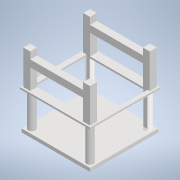
# Autodesk Inventor part: tABLE
Saved by Autodesk Inventor 2021 (Build 250183000, 183)
## iProperties
Created: 2021-06-23
Part Number: tABLE
Material: Brick, Common, Brown
Document SubType Name: Modeling
Designer: user
Density: 1.95 g/cm^3
Appearance: Default
Author: user
Autodesk Inventor part; units mm, degrees
ref_plane "YZ Plane" through (0, 0, 0) normal (1, 0, 0) x (0, 1, 0)
ref_plane "XZ Plane" through (0, 0, 0) normal (0, 1, 0) x (-1, 0, 0)
ref_plane "XY Plane" through (0, 0, 0) normal (0, 0, 1) x (1, 0, 0)
sketch "Sketch6" plane through (0, 0, 0) normal (0, 1, 0) x (-1, 0, 0)
  line L0 (-10, -10) -> (10, -10)
  line L1 (10, -10) -> (10, 10)
  line L2 (10, 10) -> (-10, 10)
  line L3 (-10, 10) -> (-10, -10)
  line L4 (-10, -10) -> (10, 10) construction
  line L5 (10, -10) -> (-10, 10) construction
  point P0 (0, 0)
  dimension "d28" = 20
  dimension "d29" = 20
  constraints: 12 end point, 2 midpoint, 2 parallel, 1 horizontal, 1 perpendicular
  measures "d28" distance of L2.end L1.end
  measures "d29" distance of L1.end L0.end
extrude "Extrusion6" add sketch "Sketch6" along normal blind 1
sketch "Sketch7" plane through (0, 1, 0) normal (0, 1, 0) x (1, 0, 0)
  circle A0 centre (-8.5, -8.5) radius 1
  line L0 (-10, 10) -> (-10, -10) projected
  line L1 (-10, -10) -> (10, -10) projected
  point P0 (0, 0)
  dimension "d32" = 2
  dimension "d33" = 0.5
  dimension "d34" = 0.5
  constraints: 1 centre point
  measures "d32" diameter of A0
  measures "d33" distance edge to line of A0 L0
  measures "d34" distance edge to line of A0 L1
extrude "Extrusion7" add sketch "Sketch7" along normal blind 10
sketch "Sketch8" plane through (0, 1, 0) normal (0, 1, 0) x (1, 0, 0)
  circle A0 centre (-8.5, 8.5) radius 1
  line L0 (-10, 10) -> (-10, -10) projected
  line L1 (10, 10) -> (-10, 10) projected
  point P0 (0, 0)
  dimension "d37" = 2
  dimension "d38" = 0.5
  dimension "d39" = 0.5
  constraints: 1 centre point
  measures "d37" diameter of A0
  measures "d38" distance edge to line of A0 L0
  measures "d39" distance edge to line of A0 L1
extrude "Extrusion8" add sketch "Sketch8" along normal blind 10
sketch "Sketch9" plane through (0, 1, 0) normal (0, 1, 0) x (1, 0, 0)
  circle A0 centre (8.5, -8.5) radius 1
  line L0 (10, -10) -> (10, 10) projected
  line L1 (-10, -10) -> (10, -10) projected
  point P0 (0, 0)
  dimension "d42" = 2
  dimension "d43" = 0.5
  dimension "d44" = 0.5
  constraints: 1 centre point
  measures "d42" diameter of A0
  measures "d43" distance edge to line of A0 L0
  measures "d44" distance edge to line of A0 L1
extrude "Extrusion9" add sketch "Sketch9" along normal blind 10
sketch "Sketch10" plane through (0, 1, 0) normal (0, 1, 0) x (1, 0, 0)
  circle A0 centre (8.5, 8.5) radius 1
  line L0 (10, -10) -> (10, 10) projected
  line L1 (10, 10) -> (-10, 10) projected
  point P0 (0, 0)
  dimension "d47" = 2
  dimension "d48" = 0.5
  dimension "d49" = 0.5
  constraints: 1 centre point
  measures "d47" diameter of A0
  measures "d48" distance edge to line of A0 L0
  measures "d49" distance edge to line of A0 L1
extrude "Extrusion10" add sketch "Sketch10" along normal blind 10
sketch "Sketch11" plane through (-8.5, 11, 8.5) normal (0, 1, 0) x (1, 0, 0)
  line L0 (18.75, 18.75) -> (-1.75, 18.75)
  line L1 (-1.75, 18.75) -> (-1.75, -1.75)
  line L2 (-1.75, -1.75) -> (18.75, -1.75)
  line L3 (18.75, -1.75) -> (18.75, 18.75)
  line L4 (18.75, 18.75) -> (-1.75, -1.75) construction
  line L5 (-1.75, 18.75) -> (18.75, -1.75) construction
  point P0 (8.5, 8.5)
  dimension "d52" = 20.5
  dimension "d53" = 20.5
  constraints: 12 end point, 2 midpoint, 2 parallel, 1 horizontal, 1 perpendicular
  measures "d52" distance of L2.end L1.end
  measures "d53" distance of L1.end L0.end
extrude "Extrusion11" add sketch "Sketch11" along normal blind 0.5
sketch "Sketch12" plane through (-8.5, 11.5, 8.5) normal (0, 1, 0) x (1, 0, 0)
  point P0 (8.5, 8.5)
sketch "Sketch13" plane through (-8.5, 11.5, 8.5) normal (0, 1, 0) x (1, 0, 0)
  line L0 (0.75, 0.75) -> (-1.25, 0.75)
  line L1 (-1.25, 0.75) -> (-1.25, -1.25)
  line L2 (-1.25, -1.25) -> (0.75, -1.25)
  line L3 (0.75, -1.25) -> (0.75, 0.75)
  line L4 (0.75, 0.75) -> (-1.25, -1.25) construction
  line L5 (-1.25, 0.75) -> (0.75, -1.25) construction
  line L6 (-1.75, -1.75) -> (18.75, -1.75) projected
  line L7 (-1.75, 18.75) -> (-1.75, -1.75) projected
  point P0 (8.5, 8.5)
  point P1 (-0.25, -0.25)
  dimension "d56" = 2
  dimension "d57" = 2
  dimension "d58" = 0.5
  dimension "d59" = 0.5
  constraints: 12 end point, 2 midpoint, 2 parallel, 1 horizontal, 1 perpendicular
  measures "d56" distance of L2.end L1.end
  measures "d57" distance of L1.end L0.end
  measures "d58" distance between parallel lines of L2 L6
  measures "d59" distance between parallel lines of L1 L7
extrude "Extrusion12" add sketch "Sketch13" along normal blind 10
sketch "Sketch14" plane through (-8.5, 11.5, 8.5) normal (0, 1, 0) x (1, 0, 0)
  line L0 (-1.25, 16.25) -> (0.75, 16.25)
  line L1 (0.75, 16.25) -> (0.75, 18.25)
  line L2 (0.75, 18.25) -> (-1.25, 18.25)
  line L3 (-1.25, 18.25) -> (-1.25, 16.25)
  line L4 (-1.25, 16.25) -> (0.75, 18.25) construction
  line L5 (0.75, 16.25) -> (-1.25, 18.25) construction
  line L6 (-1.75, 18.75) -> (-1.75, -1.75) projected
  line L7 (18.75, 18.75) -> (-1.75, 18.75) projected
  point P0 (8.5, 8.5)
  point P1 (-0.25, 17.25)
  dimension "d62" = 2
  dimension "d63" = 2
  dimension "d64" = 0.5
  dimension "d65" = 0.5
  constraints: 12 end point, 2 midpoint, 2 parallel, 1 horizontal, 1 perpendicular
  measures "d62" distance of L2.end L1.end
  measures "d63" distance of L1.end L0.end
  measures "d64" distance between parallel lines of L3 L6
  measures "d65" distance between parallel lines of L2 L7
extrude "Extrusion13" add sketch "Sketch14" along normal blind 10
sketch "Sketch15" plane through (-8.5, 11.5, 8.5) normal (0, 1, 0) x (1, 0, 0)
  line L0 (18.25, 0.75) -> (16.25, 0.75)
  line L1 (16.25, 0.75) -> (16.25, -1.25)
  line L2 (16.25, -1.25) -> (18.25, -1.25)
  line L3 (18.25, -1.25) -> (18.25, 0.75)
  line L4 (18.25, 0.75) -> (16.25, -1.25) construction
  line L5 (16.25, 0.75) -> (18.25, -1.25) construction
  line L6 (-1.75, -1.75) -> (18.75, -1.75) projected
  line L7 (18.75, -1.75) -> (18.75, 18.75) projected
  point P0 (8.5, 8.5)
  point P1 (17.25, -0.25)
  dimension "d68" = 2
  dimension "d69" = 2
  dimension "d70" = 0.5
  dimension "d71" = 0.5
  constraints: 12 end point, 2 midpoint, 2 parallel, 1 horizontal, 1 perpendicular
  measures "d68" distance of L2.end L1.end
  measures "d69" distance of L1.end L0.end
  measures "d70" distance between parallel lines of L2 L6
  measures "d71" distance between parallel lines of L3 L7
extrude "Extrusion14" add sketch "Sketch15" along normal blind 10
sketch "Sketch16" plane through (-8.5, 11.5, 8.5) normal (0, 1, 0) x (1, 0, 0)
  line L0 (16.25, 16.25) -> (18.25, 16.25)
  line L1 (18.25, 16.25) -> (18.25, 18.25)
  line L2 (18.25, 18.25) -> (16.25, 18.25)
  line L3 (16.25, 18.25) -> (16.25, 16.25)
  line L4 (16.25, 16.25) -> (18.25, 18.25) construction
  line L5 (18.25, 16.25) -> (16.25, 18.25) construction
  line L6 (18.75, -1.75) -> (18.75, 18.75) projected
  line L7 (18.75, 18.75) -> (-1.75, 18.75) projected
  point P0 (8.5, 8.5)
  point P1 (17.25, 17.25)
  dimension "d74" = 2
  dimension "d75" = 2
  dimension "d76" = 0.5
  dimension "d77" = 0.5
  constraints: 12 end point, 2 midpoint, 2 parallel, 1 horizontal, 1 perpendicular
  measures "d74" distance of L2.end L1.end
  measures "d75" distance of L1.end L0.end
  measures "d76" distance between parallel lines of L1 L6
  measures "d77" distance between parallel lines of L2 L7
extrude "Extrusion15" add sketch "Sketch16" along normal blind 10
sketch "Sketch17" plane through (-8.5, 11.5, 8.5) normal (0, 1, 0) x (1, 0, 0)
  line L0 (-1.25, 0.75) -> (0.75, 0.75) projected
  line L1 (-0.25, 0.75) -> (17.5992, 0.75)
  line L2 (17.5992, 0.75) -> (17.5992, 16.25)
  line L3 (17.5992, 16.25) -> (-0.25, 16.25)
  line L4 (-0.25, 16.25) -> (-0.25, 0.75)
  point P0 (8.5, 8.5)
  constraints: 8 end point, 2 parallel, 1 horizontal, 1 midpoint, 1 perpendicular
extrude "Extrusion16" cut sketch "Sketch17" against normal blind 10
sketch "Sketch18" plane through (7.75, 11.5, -9.75) normal (-1, 0, 0) x (0, 0, 1)
  point P0 (9.75, -11.5)
sketch "Sketch19" plane through (7.75, 11.5, -9.75) normal (-1, 0, 0) x (0, 0, 1)
  point P0 (9.75, -11.5)
sketch "Sketch20" plane through (7.75, 11.5, -9.75) normal (-1, 0, 0) x (0, 0, 1)
  point P0 (9.75, -11.5)
sketch "Sketch21" plane through (7.75, 11.5, -9.75) normal (-1, 0, 0) x (0, 0, 1)
  line L0 (2, 8) -> (0, 8)
  line L1 (0, 8) -> (0, 6)
  line L2 (0, 6) -> (2, 6)
  line L3 (2, 6) -> (2, 8)
  line L4 (2, 0) -> (2, 10) projected
  line L5 (0, 10) -> (2, 10) projected
  point P0 (9.75, -11.5)
  dimension "d82" = 2
  dimension "d83" = 2
  dimension "d84" = 0
  dimension "d85" = 2
  constraints: 8 end point, 2 parallel, 1 horizontal, 1 perpendicular
  measures "d82" distance of L2.end L1.end
  measures "d83" distance of L1.end L0.end
  measures "d84" distance between parallel lines of L3 L4
  measures "d85" distance between parallel lines of L5 L0
extrude "Extrusion17" add sketch "Sketch21" along normal blind 16
sketch "Sketch22" plane through (7.75, 11.5, 7.75) normal (-1, 0, 0) x (0, 0, 1)
  line L0 (2, 8) -> (0, 8)
  line L1 (0, 8) -> (0, 6)
  line L2 (0, 6) -> (2, 6)
  line L3 (2, 6) -> (2, 8)
  line L4 (2, 0) -> (2, 10) projected
  line L5 (0, 10) -> (2, 10) projected
  point P0 (-7.75, -11.5)
  dimension "d88" = 2
  dimension "d89" = 2
  dimension "d90" = 0
  dimension "d91" = 2
  constraints: 8 end point, 2 parallel, 1 horizontal, 1 perpendicular
  measures "d88" distance of L2.end L1.end
  measures "d89" distance of L1.end L0.end
  measures "d90" distance between parallel lines of L3 L4
  measures "d91" distance between parallel lines of L0 L5
extrude "Extrusion18" add sketch "Sketch22" along normal blind 16
sketch "Sketch23" plane through (0, 0, 0) normal (0, -1, 0) x (1, 0, 0)
  circle A0 centre (0, 0) radius 0.5
  dimension "d94" = 1
  constraints: 1 centre point, 1 coincident
  measures "d94" diameter of A0
extrude "Extrusion19" cut sketch "Sketch23" against normal blind 1
body "Solid2"
